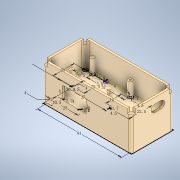
# Autodesk Inventor part: 外壳
Saved by Autodesk Inventor 2022 (Build 260153000, 153)
## iProperties
Created: 2022-08-05
Part Number: 外壳
Material: 聚乙烯，高密度
Document SubType Name: Modeling
Designer: Shane
Density: 0.952 g/cm^3
Appearance: 平滑 - 灰白色
Author: Shane
Autodesk Inventor part; units mm, degrees
ref_plane "YZ Plane" through (0, 0, 0) normal (1, 0, 0) x (0, 1, 0)
ref_plane "XZ Plane" through (0, 0, 0) normal (0, 1, 0) x (-1, 0, 0)
ref_plane "XY Plane" through (0, 0, 0) normal (0, 0, 1) x (1, 0, 0)
sketch "草图1" plane through (0, 0, 0) normal (0, 1, 0) x (-1, 0, 0)
  line L0 (4, 0) -> (21, 0)
  line L1 (25, 4) -> (25, 26)
  line L2 (21, 30) -> (4, 30)
  line L3 (0, 26) -> (0, 4)
  arc A0 (25, 26) -> (21, 30) centre (21, 26) ccw
  arc A1 (4, 30) -> (0, 26) centre (4, 26) ccw
  arc A2 (0, 4) -> (4, 0) centre (4, 4) ccw
  arc A3 (21, 0) -> (25, 4) centre (21, 4) ccw
  circle A4 centre (21, 26) radius 1.1
  circle A5 centre (4, 26) radius 1.1
  line L4 (25, 26) -> (25, 36.5)
  line L5 (25, 36.5) -> (-56, 36.5)
  line L6 (-56, 36.5) -> (-56, 0)
  line L7 (-56, 0) -> (21, 0)
  circle A6 centre (4, 26) radius 2
  circle A7 centre (21, 26) radius 2
  line L8 (27, 39.5) -> (27, 38.5)
  line L9 (27, 38.5) -> (-58, 38.5)
  line L10 (-58, 38.5) -> (-58, -2)
  line L11 (-58, -2) -> (22.5, -2)
  line L12 (27, 39.5) -> (27, -2)
  line L13 (27, -2) -> (22.5, -2)
  point P0 (0, 0)
  point P1 (25, 30)
  point P2 (25, 0)
  point P3 (0, 30)
  point P4 (4, 0)
  point P5 (27, 38.5)
  dimension "d120" = 12
  dimension "d121" = 0
  dimension "d0" = 25
  dimension "d1" = 30
  dimension "d2" = 4
  dimension "d3" = 2.2
  dimension "d4" = 2.2
  dimension "d5" = 10.5
  dimension "d6" = 81
  dimension "d9" = 4
  dimension "d10" = 4
  dimension "d13" = 2
  constraints: 28 end point, 9 tangent, 8 centre point, 8 perpendicular, 8 point on circle, 8 point on line, 4 coincident, 3 equal radius, 2 parallel, 2 vertical, 1 horizontal, 3 other
  measures "d0" distance of point (0, 30) point (25, 30)
  measures "d1" distance of point (25, 30) point (25, 0)
  measures "d2" radius of A0
  measures "d3" diameter of A4
  measures "d4" diameter of A5
  measures "d5" distance of L1.end L4.end
  measures "d6" distance of L4.end L5.end
  measures "d9" diameter of A6
  measures "d10" diameter of A7
  measures "d13" distance between parallel lines of L4 L8
extrude "拉伸1" add sketch "草图1" along normal blind 12 contours A2 L3 A1 L2 A0 L1 A3 L0 | L7 L6 L5 L4 A0 L2 A1 L3 A2 | A6 | A7
extrude "拉伸3" add sketch "草图1" along normal blind 36 contours L12 L13 L11 L10 L9
sketch "草图2" plane through (0, 12, 0) normal (0, 1, 0) x (1, 0, 0)
  circle A0 centre (-22.5, -2.5) radius 2
  circle A1 centre (-2.5, -2.5) radius 2
  line L0 (-25, -36.5) -> (-25, -4) projected
  line L1 (-21, 0) -> (56, 0) projected
  line L2 (-22.5, -2.5) -> (-2.5, -2.5)
  point P0 (0, 0)
  dimension "d16" = 4
  dimension "d17" = 4
  dimension "d18" = 2.5
  dimension "d19" = 2.5
  dimension "d20" = 2.5
  constraints: 2 centre point, 2 end point
  measures "d16" diameter of A0
  measures "d17" diameter of A1
  measures "d18" distance from line of L0 L2.start
  measures "d19" distance from line of L1 L2.start
  measures "d20" distance from line of L1 L2.end
sketch "草图4" plane through (-27, 0, 38.5) normal (0, 0, 1) x (1, 0, 0)
  line L0 (19, 24.5) -> (41.5, 24.5)
  line L1 (41.5, 24.5) -> (41.5, 12)
  line L2 (41.5, 12) -> (19, 12)
  line L3 (19, 12) -> (19, 24.5)
  line L4 (0, 0) -> (85, 0) projected
  line L5 (85, 0) -> (85, 36) projected
  circle A0 centre (16.35, 18.25) radius 0.85
  circle A1 centre (44.15, 18.25) radius 0.85
  line L6 (30.25, 24.5) -> (30.25, 12)
  line L7 (2, 12) -> (83, 12) projected
  line L8 (40.2, 20.05) -> (42.8, 20.05)
  line L9 (42.8, 20.05) -> (42.8, 16.45)
  line L10 (42.8, 16.45) -> (40.2, 16.45)
  line L11 (40.2, 16.45) -> (40.2, 20.05)
  line L12 (40.2, 20.05) -> (42.8, 16.45) construction
  line L13 (42.8, 20.05) -> (40.2, 16.45) construction
  point P0 (27, 0)
  point P1 (41.5, 18.25)
  point P2 (41.5, 20.05)
  point P3 (41.5, 16.45)
  dimension "d27" = 22.5
  dimension "d28" = 12.5
  dimension "d29" = 12
  dimension "d30" = 43.5
  dimension "d31" = 13.9
  dimension "d32" = 13.9
  dimension "d33" = 6.25
  dimension "d34" = 6.25
  dimension "d35" = 1.7
  dimension "d36" = 1.7
  dimension "d118" = 2.6
  dimension "d119" = 3.6
  constraints: 22 end point, 4 midpoint, 4 parallel, 3 perpendicular, 2 centre point, 2 horizontal, 1 point on line
  measures "d27" distance of L1.end L2.end
  measures "d28" distance of L0.end L1.end
  measures "d29" distance between parallel lines of L4 L2
  measures "d30" distance between parallel lines of L5 L1
  measures "d31" distance from line of L6 A0.centre
  measures "d32" distance from line of L6 A1.centre
  measures "d33" distance from line of L2 A0.centre
  measures "d34" distance from line of L2 A1.centre
  measures "d35" diameter of A0
  measures "d36" diameter of A1
  measures "d118" distance of L9.end L10.end
  measures "d119" distance of L8.end L9.end
extrude "拉伸6" cut sketch "草图4" against normal blind 2
sketch "草图6" plane through (0, 12, 0) normal (0, 1, 0) x (1, 0, 0)
  circle A0 centre (-15.5, -22.5) radius 2
  circle A1 centre (-22.5, -2.5) radius 2 projected
  line L0 (-25, -36.5) -> (-25, -4) projected
  circle A2 centre (-15.5, -2.5) radius 2
  line L1 (-21, 0) -> (56, 0) projected
  circle A3 centre (21.5, -22.5) radius 2.25
  circle A4 centre (21.4966, -3) radius 2.25
  circle A5 centre (21.5, -22.5) radius 0.85
  circle A6 centre (21.4966, -3) radius 0.85
  point P0 (0, 0)
  dimension "d51" = 9.5
  dimension "d52" = 4
  dimension "d53" = 4
  dimension "d54" = 20
  dimension "d55" = 22.5
  dimension "d56" = 9.5
  dimension "d57" = 4.5
  dimension "d58" = 37
  dimension "d59" = 22.5
  dimension "d60" = 4.5
  dimension "d61" = 15
  dimension "d62" = 37
  dimension "d63" = 1.7
  dimension "d64" = 1.7
  constraints: 6 centre point, 2 coincident
  measures "d51" distance from line of L0 A0.centre
  measures "d52" diameter of A2
  measures "d53" diameter of A0
  measures "d54" distance of A0.centre A2.centre
  measures "d55" distance from line of L1 A0.centre
  measures "d56" distance from line of L0 A2.centre
  measures "d57" diameter of A3
  measures "d58" distance of A0.centre A3.centre
  measures "d59" distance from line of L1 A3.centre
  measures "d60" diameter of A4
  measures "d62" distance of A2.centre A4.centre
  measures "d63" diameter of A5
  measures "d64" diameter of A6
extrude "拉伸8" add sketch "草图6" along normal blind 14 contours A0 | A2 | A3 | A4
extrude "拉伸9" add sketch "草图1" along normal blind 12 contours A4 | A5
extrude "拉伸10" cut sketch "草图6" against normal blind 12 contours A5 | A6
fillet "圆角1" radius 4 3 edges at (-25, 24, 36.5) (56, 24, 36.5) (56, 24, 0)
fillet "圆角2" radius 2.5 2 edges at (-27, 18, -2) (-27, 18, 38.5)
fillet "圆角3" radius 2.5 2 edges at (58, 18, 38.5) (58, 18, -2)
sketch "草图11" plane through (0, 36, 0) normal (0, 1, 0) x (1, 0, 0)
  circle A0 centre (-25, 0) radius 1
  line L0 (-27, -0.5) -> (-27, -36) projected
  line L1 (-25, -4) -> (-25, -32.5) projected
  line L2 (55.5, 2) -> (-24.5, 2) projected
  circle A1 centre (-25, -36.5) radius 1
  line L3 (-24.5, -38.5) -> (55.5, -38.5) projected
  circle A2 centre (56, -36.5) radius 1
  line L4 (58, -36) -> (58, -0.5) projected
  circle A3 centre (56, 0) radius 1
  line L5 (-23, -38.5) -> (-27, -38.5)
  line L6 (-27, -38.5) -> (-27, -34.5)
  line L7 (-27, -34.5) -> (-23, -34.5)
  line L8 (-23, -34.5) -> (-23, -38.5)
  line L9 (-23, -38.5) -> (-27, -34.5) construction
  line L10 (-27, -38.5) -> (-23, -34.5) construction
  line L11 (-23, 2) -> (-27, 2)
  line L12 (-27, 2) -> (-27, -2)
  line L13 (-27, -2) -> (-23, -2)
  line L14 (-23, -2) -> (-23, 2)
  line L15 (-23, 2) -> (-27, -2) construction
  line L16 (-27, 2) -> (-23, -2) construction
  line L17 (54, -2) -> (58, -2)
  line L18 (58, -2) -> (58, 2)
  line L19 (58, 2) -> (54, 2)
  line L20 (54, 2) -> (54, -2)
  line L21 (54, -2) -> (58, 2) construction
  line L22 (58, -2) -> (54, 2) construction
  line L23 (54, -38.5) -> (58, -38.5)
  line L24 (58, -38.5) -> (58, -34.5)
  line L25 (58, -34.5) -> (54, -34.5)
  line L26 (54, -34.5) -> (54, -38.5)
  line L27 (54, -38.5) -> (58, -34.5) construction
  line L28 (58, -38.5) -> (54, -34.5) construction
  point P0 (0, 0)
  point P1 (55.5, -38.5)
  point P2 (-24.5, -48.5)
  point P3 (55.5, -38.5)
  dimension "d90" = 2
  dimension "d91" = 2
  dimension "d92" = 2
  dimension "d93" = 2
  dimension "d94" = 2
  dimension "d95" = 2
  dimension "d96" = 2
  dimension "d97" = 2
  dimension "d98" = 2
  dimension "d99" = 2
  dimension "d100" = 2
  dimension "d101" = 2
  dimension "d111" = 4
  dimension "d112" = 4
  dimension "d113" = 4
  dimension "d114" = 4
  dimension "d115" = 4
  dimension "d116" = 4
  dimension "d117" = 4
  constraints: 48 end point, 8 midpoint, 8 parallel, 4 centre point, 4 horizontal, 4 perpendicular, 1 point on line, 1 other
  measures "d90" diameter of A0
  measures "d91" distance from line of L0 A0.centre
  measures "d92" distance from line of L2 A0.centre
  measures "d93" diameter of A1
  measures "d94" distance from line of L0 A1.centre
  measures "d96" diameter of A2
  measures "d97" distance from line of L4 A2.centre
  measures "d99" diameter of A3
  measures "d100" distance from line of L2 A3.centre
  measures "d101" distance from line of L4 A3.centre
  measures "d111" distance of L5.end L6.end
  measures "d112" distance of L12.end L11.end
  measures "d113" distance of L6.end L7.end
  measures "d114" distance of L19.end L18.end
  measures "d115" distance of L18.end L17.end
  measures "d116" distance of L25.end L24.end
  measures "d117" distance of L24.end L23.end
extrude "拉伸14" cut sketch "草图11" against normal blind 4 contours A0 | L12 L11 L2 L14 L13 L0 | L7 L8 L3 L5 L6 L0 | L2 L19 L18 L4 L17 L20 | L26 L25 L4 L24 L23 L3 | A1 | A2 | A3
sketch "草图12" plane through (58, 0, 36) normal (1, 0, 0) x (0, 0, -1)
  line L0 (15.0264, 27) -> (28.4358, 27)
  line L1 (0, 0) -> (35.5, 0) projected
  line L2 (23, 0) -> (23, 34.6188)
  line L3 (35.5, 36) -> (35.5, 0) projected
  line L4 (20, 30.5) -> (26, 30.5)
  line L5 (29.5, 27) -> (29.5, 27)
  line L6 (26, 23.5) -> (20, 23.5)
  line L7 (16.5, 27) -> (16.5, 27)
  line L8 (16.5, 30.5) -> (29.5, 23.5) construction
  line L9 (29.5, 30.5) -> (16.5, 23.5) construction
  arc A0 (20, 30.5) -> (16.5, 27) centre (20, 27) ccw
  arc A1 (16.5, 27) -> (20, 23.5) centre (20, 27) ccw
  arc A2 (26, 23.5) -> (29.5, 27) centre (26, 27) ccw
  arc A3 (29.5, 27) -> (26, 30.5) centre (26, 27) ccw
  point P0 (36, 0)
  point P1 (23, 27)
  point P2 (16.5, 27)
  dimension "d104" = 27
  dimension "d105" = 12.5
  dimension "d106" = 13
  dimension "d107" = 7
  dimension "d108" = 3.5
  constraints: 16 end point, 11 point on line, 8 point on circle, 8 tangent, 4 centre point, 3 equal radius, 2 horizontal, 2 midpoint, 2 parallel, 1 perpendicular, 1 vertical
  measures "d104" distance between parallel lines of L1 L0
  measures "d105" distance between parallel lines of L3 L2
  measures "d106" distance of L8.end L9.end
  measures "d107" distance of L9.start L8.end
  measures "d108" radius of A0
extrude "拉伸15" cut sketch "草图12" against normal blind 2
sketch "草图13" plane through (0, 0, 0) normal (0, -1, 0) x (1, 0, 0)
  circle A0 centre (21.5, 22.5) radius 0.85 projected
  circle A1 centre (21.5, 22.5) radius 0.85
  circle A2 centre (21.4966, 3) radius 0.85 projected
  circle A3 centre (21.4966, 3) radius 0.85
  point P0 (0, 0)
  constraints: 2 centre point, 2 coincident
extrude "拉伸16" add sketch "草图13" against normal blind 12
